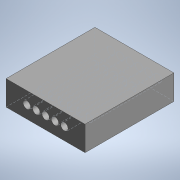
# Autodesk Inventor part: Single_Mode_Pan
Saved by Autodesk Inventor 2021 (Build 250183000, 183)
## iProperties
Part Number: Single_Mode_Pan
Material: Generic
Document SubType Name: Modeling
Designer: Vatsan
Appearance: Default
Author: Vatsan
Autodesk Inventor part; units mm, degrees
ref_plane "YZ Plane" through (0, 0, 0) normal (1, 0, 0) x (0, 1, 0)
ref_plane "XZ Plane" through (0, 0, 0) normal (0, 1, 0) x (-1, 0, 0)
ref_plane "XY Plane" through (0, 0, 0) normal (0, 0, 1) x (1, 0, 0)
sketch "Sketch1" plane through (0, 0, 0) normal (0, 0, 1) x (1, 0, 0)
  line L0 (0, 0) -> (-50.8, 0)
  line L1 (-50.8, 0) -> (-50.8, 15.875)
  line L2 (-50.8, 15.875) -> (0, 15.875)
  line L3 (0, 15.875) -> (0, 0)
  point P0 (-10.2858, 7.9375)
  point P1 (-16.3182, 7.9375)
  point P2 (-22.3507, 7.9375)
  point P3 (-28.3832, 7.9375)
  point P4 (-34.4157, 7.9375)
  point P5 (-40.4482, 7.9375)
  constraints: 8 end point
sketch "Sketch2" plane through (0, 0, 57.15) normal (0, 0, 1) x (1, 0, 0)
  point P0 (-13.302, 7.9375)
  point P1 (-19.3345, 7.9375)
  point P2 (-25.367, 7.9375)
  point P3 (-31.3995, 7.9375)
  point P4 (-37.432, 7.9375)
extrude "Extrusion1" add sketch "Sketch1" along normal blind 57.15
hole "Hole1" at (-10.2858, 7.9375, 0) at (-16.3182, 7.9375, 0) at (-22.3507, 7.9375, 0) at (-28.3832, 7.9375, 0) at (-34.4157, 7.9375, 0) at (-40.4482, 7.9375, 0) direction (0, 0, 1) diameter 4.7625 depth 44.4995 tip angle 118
hole "Hole2" at (-13.302, 7.9375, 57.15) at (-19.3345, 7.9375, 57.15) at (-25.367, 7.9375, 57.15) at (-31.3995, 7.9375, 57.15) at (-37.432, 7.9375, 57.15) direction (0, 0, -1) diameter 4.7625 depth 44.4995 tip angle 118
body "Solid1"
